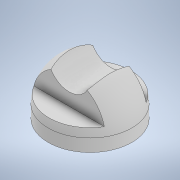
# Autodesk Inventor part: Part4
Saved by Autodesk Inventor 2022 (Build 260153000, 153)
## iProperties
Created: 2022-01-07
Part Number: Part4
Material: Generic
Document SubType Name: Modeling
Designer: nguye
Density: 1 g/cm^3
Appearance: Default
Author: nguye
Autodesk Inventor part; units mm, degrees
ref_plane "YZ Plane" through (0, 0, 0) normal (1, 0, 0) x (0, 1, 0)
ref_plane "XZ Plane" through (0, 0, 0) normal (0, 1, 0) x (-1, 0, 0)
ref_plane "XY Plane" through (0, 0, 0) normal (0, 0, 1) x (1, 0, 0)
sketch "Sketch1" plane through (0, 0, 0) normal (0, 1, 0) x (-1, 0, 0)
  circle A0 centre (0, 0) radius 100
  dimension "d0" = 200
  constraints: 1 centre point, 1 coincident
  measures "d0" diameter of A0
extrude "Extrusion1" add sketch "Sketch1" along normal blind 130
fillet "Fillet1" radius 100 1 edges at (100, 130, 0)
sketch "Sketch2" plane through (0, 0, 0) normal (0, 0, 1) x (1, 0, 0)
  circle A0 centre (0, 130) radius 50
  point P0 (0, 0)
  dimension "d5" = 100
  constraints: 1 centre point
  measures "d5" diameter of A0
extrude "Extrusion2" cut sketch "Sketch2" along normal mid plane 200
sketch "Sketch3" plane through (0, 0, 0) normal (1, 0, 0) x (0, 1, 0)
  line L0 (30, -100) -> (30, 100) projected
  line L1 (50, -100) -> (110.476, -100)
  line L2 (110.476, -100) -> (110.476, -50)
  line L3 (110.476, -50) -> (50, -50)
  line L4 (50, -50) -> (50, -100)
  line L5 (0, 100) -> (30, 100) projected
  line L6 (50, 100) -> (110.476, 100)
  line L7 (110.476, 100) -> (110.476, 50)
  line L8 (110.476, 50) -> (50, 50)
  line L9 (50, 50) -> (50, 100)
  point P0 (0, 0)
  point P1 (30, 100)
  dimension "d8" = 20
  dimension "d9" = 50
  dimension "d10" = 20
  dimension "d11" = 50
  constraints: 16 end point, 4 parallel, 2 horizontal, 2 perpendicular
  measures "d8" distance of L0.start L1.start
  measures "d9" distance of L2.end L1.end
  measures "d10" distance of point (30, 100) L6.start
  measures "d11" distance of L6.end L7.end
extrude "Extrusion3" cut sketch "Sketch3" along normal mid plane 200
body "Solid1"
